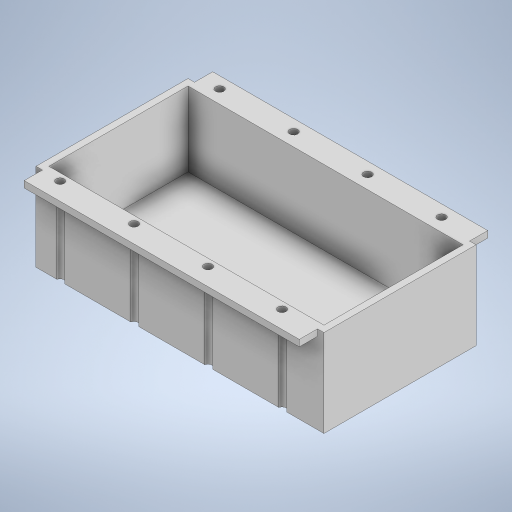
# Autodesk Inventor part: pruebabateria
Saved by Autodesk Inventor 2024.3 (Build 283343000, 343)
## iProperties
Created: 2025-10-08
Part Number: pruebabateria
Material: Generic
Document SubType Name: Modeling
Designer: jscme
Density: 1 g/cm^3
Appearance: Default
Author: jscme
Autodesk Inventor part; units mm, degrees
ref_plane "YZ Plane" through (0, 0, 0) normal (1, 0, 0) x (0, 1, 0)
ref_plane "XZ Plane" through (0, 0, 0) normal (0, 1, 0) x (-1, 0, 0)
ref_plane "XY Plane" through (0, 0, 0) normal (0, 0, 1) x (1, 0, 0)
sketch "Sketch1" plane through (0, 0, 0) normal (0, 1, 0) x (-1, 0, 0)
  line L0 (42.5, 21.5) -> (-42.5, 21.5)
  line L1 (-42.5, 21.5) -> (-42.5, -21.5)
  line L2 (-42.5, -21.5) -> (42.5, -21.5)
  line L3 (42.5, -21.5) -> (42.5, 21.5)
  point P0 (0, 0)
  point P1 (0, -21.5)
  point P2 (42.5, 0)
  dimension "d0" = 43
  dimension "d1" = 85
  constraints: 8 end point, 2 midpoint, 2 parallel, 1 horizontal, 1 horizontal alignment, 1 perpendicular, 1 vertical alignment
  measures "d0" distance of L0.end L1.end
  measures "d1" distance of L1.end L2.end
extrude "Extrusion1" add sketch "Sketch1" along normal blind 4
sketch "Sketch2" plane through (-42.5, 0, 21.5) normal (0, 0, 1) x (1, 0, 0)
  line L0 (0, 25) -> (85, 25)
  line L1 (85, 25) -> (85, 0)
  line L2 (85, 0) -> (0, 0)
  line L3 (0, 0) -> (0, 25)
  point P0 (42.5, 0)
  dimension "d4" = 25
  constraints: 8 end point, 2 parallel, 1 horizontal, 1 perpendicular
  measures "d4" distance of L0.end L1.end
extrude "Extrusion2" add sketch "Sketch2" along normal blind 2
sketch "Sketch3" plane through (42.5, 0, -21.5) normal (0, 0, -1) x (-1, 0, 0)
  line L0 (0, 25) -> (85, 25) projected
  line L1 (0, 0) -> (85, 0) projected
  line L2 (0, 25) -> (85, 25)
  line L3 (85, 25) -> (85, 0)
  line L4 (85, 0) -> (0, 0)
  line L5 (0, 0) -> (0, 25)
  point P0 (42.5, 0)
  constraints: 8 end point, 2 parallel, 1 horizontal, 1 perpendicular
extrude "Extrusion3" add sketch "Sketch3" along normal blind 2
sketch "Sketch4" plane through (-42.5, 25, -21.5) normal (0, 1, 0) x (1, 0, 0)
  line L0 (0, -45) -> (0, 2) projected
  line L1 (0, 7.62) -> (85, 7.62)
  line L2 (85, 7.62) -> (85, 0)
  line L3 (85, 0) -> (0, 0)
  line L4 (0, 0) -> (0, 7.62)
  point P0 (42.5, -21.5)
  point P1 (85, 3.81)
  point P2 (85, 2)
  dimension "d15" = 7.62
  constraints: 8 end point, 2 parallel, 1 horizontal, 1 midpoint, 1 perpendicular, 1 point on line, 1 vertical alignment
  measures "d15" distance between parallel lines of L3 L1
extrude "Extrusion4" add sketch "Sketch4" along normal blind 2
sketch "Sketch5" plane through (-42.5, 25, 21.5) normal (0, 1, 0) x (1, 0, 0)
  line L0 (0, -2) -> (0, 45) projected
  line L1 (0, 0) -> (85, 0)
  line L2 (85, 0) -> (85, -7.62)
  line L3 (85, -7.62) -> (0, -7.62)
  line L4 (0, -7.62) -> (0, 0)
  line L5 (85, 0) -> (85, -2) projected
  line L6 (85, 0) -> (0, 0) projected
  point P0 (42.5, 21.5)
  point P1 (85, -3.81)
  point P2 (85, -1)
  point P3 (42.5, 0)
  dimension "d17" = 7.62
  constraints: 8 end point, 4 midpoint, 2 parallel, 1 horizontal, 1 perpendicular, 1 point on line, 1 vertical alignment
  measures "d17" distance between parallel lines of L3 L1
extrude "Extrusion5" add sketch "Sketch5" along normal blind 2
sketch "Sketch6" plane through (42.5, 0, 23.5) normal (1, 0, 0) x (0, 0, -1)
  line L0 (-5.62, 27) -> (2, 27) projected
  line L1 (47, 0) -> (47, 25) projected
  line L2 (0, 27) -> (47, 27)
  line L3 (47, 27) -> (47, 0)
  line L4 (47, 0) -> (0, 0)
  line L5 (0, 0) -> (0, 27)
  line L6 (0, 0) -> (0, 25) projected
  point P0 (23.5, 0)
  point P1 (0, 13.5)
  constraints: 8 end point, 2 parallel, 2 point on line, 1 horizontal, 1 midpoint, 1 perpendicular
extrude "Extrusion6" add sketch "Sketch6" along normal blind 2
sketch "Sketch7" plane through (-42.5, 0, -23.5) normal (-1, 0, 0) x (0, 0, 1)
  line L0 (-5.62, 27) -> (2, 27) projected
  line L1 (47, 25) -> (47, 0) projected
  line L2 (0, 27) -> (47, 27)
  line L3 (47, 27) -> (47, 0)
  line L4 (47, 0) -> (0, 0)
  line L5 (0, 0) -> (0, 27)
  line L6 (0, 0) -> (0, 25) projected
  point P0 (23.5, 0)
  point P1 (0, 12.5)
  constraints: 8 end point, 2 parallel, 2 point on line, 1 horizontal, 1 midpoint, 1 perpendicular
extrude "Extrusion7" add sketch "Sketch7" along normal blind 2
sketch "Sketch8" plane through (-42.5, 27, -21.5) normal (0, 1, 0) x (1, 0, 0)
  circle A0 centre (74.2833, 4.064) radius 1.27
  line L0 (0, 0) -> (85, 0) projected
  circle A1 centre (51.4233, 4.064) radius 1.27
  circle A2 centre (28.5633, 4.064) radius 1.27
  circle A3 centre (5.7033, 4.064) radius 1.27
  line L1 (95.5719, -20.5867) -> (-13.3282, -20.5867)
  circle A4 centre (74.2833, -45.2374) radius 1.27
  circle A5 centre (51.4233, -45.2374) radius 1.27
  circle A6 centre (28.5633, -45.2374) radius 1.27
  circle A7 centre (5.7033, -45.2374) radius 1.27
  point P0 (42.5, -21.5)
  dimension "d23" = 2.54
  dimension "d24" = 4.064
  dimension "d27" = 22.86
  dimension "d34" = 49.3014
  constraints: 8 centre point, 4 symmetric about line, 2 end point, 2 horizontal, 10 other
  measures "d23" diameter of A0
  measures "d24" distance from line of L0 A0.centre
  measures "d27" distance of A0.centre A1.centre
  measures "d34" distance of A5.centre A1.centre
extrude "Extrusion8" cut sketch "Sketch8" against normal through all
body "Solid1"
